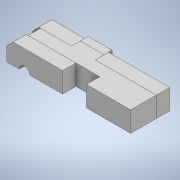
# Autodesk Inventor part: Деталь1
Saved by Autodesk Inventor 2022 (Build 260153000, 153)
## iProperties
Created: 2024-04-16
Part Number: Деталь1
Material: Типовые
Document SubType Name: Modeling
Designer: Pavel
Density: 1 g/cm^3
Appearance: По умолчанию
Mass: 255.555 g
Surface Area: 533.619 cm^2
Volume: 255.555 cm^3
Author: Pavel
Autodesk Inventor part; units mm, degrees
ref_plane "YZ Plane" through (0, 0, 0) normal (1, 0, 0) x (0, 1, 0)
ref_plane "XZ Plane" through (0, 0, 0) normal (0, 1, 0) x (-1, 0, 0)
ref_plane "XY Plane" through (0, 0, 0) normal (0, 0, 1) x (1, 0, 0)
sketch "Эскиз1" plane through (0, 0, 0) normal (0, 1, 0) x (-1, 0, 0)
  line L0 (0, 0) -> (140, 0)
  line L1 (140, 0) -> (140, 46)
  line L2 (140, 46) -> (0, 46)
  line L3 (0, 46) -> (0, 0)
  dimension "d0" = 140
  dimension "d1" = 46
  constraints: 8 end point, 2 parallel, 1 horizontal, 1 perpendicular
  measures "d0" distance of L2.end L1.end
  measures "d1" distance of L1.end L0.end
extrude "Выдавливание1" add sketch "Эскиз1" along normal blind 44
sketch "Эскиз2" plane through (0, 0, 0) normal (0, 0, -1) x (-1, 0, 0)
  line L0 (0, 44) -> (140, 44) projected
  line L1 (0, 44) -> (69, 44)
  line L2 (69, 44) -> (69, 29)
  line L3 (69, 29) -> (0, 29)
  line L4 (0, 29) -> (0, 44)
  point P0 (0, 0)
  dimension "d4" = 69
  dimension "d5" = 15
  constraints: 8 end point, 2 parallel, 1 horizontal, 1 perpendicular
  measures "d4" distance of L2.end L3.end
  measures "d5" distance of L1.end L2.end
split body "Разделение1" sketch "Эскиз2" result two bodies curves L3 L4 L1 L2 first body at (-46.6667, 0.5, 30.6667)
sketch "Эскиз3" plane through (0, 0, 0) normal (0, 0, -1) x (-1, 0, 0)
  line L0 (140, 44) -> (96, 44)
  line L1 (96, 44) -> (96, 29)
  line L2 (96, 29) -> (140, 29)
  line L3 (140, 29) -> (140, 44)
  line L4 (140, 0) -> (77, 0)
  line L5 (77, 0) -> (77, 15)
  line L6 (77, 15) -> (140, 15)
  line L7 (140, 15) -> (140, 0)
  line L8 (77, 0) -> (50, 0)
  line L9 (50, 0) -> (50, 15)
  line L10 (50, 15) -> (77, 15)
  line L11 (77, 15) -> (77, 0)
  point P0 (0, 0)
  dimension "d6" = 44
  dimension "d7" = 15
  dimension "d8" = 63
  dimension "d9" = 15
  dimension "d10" = 27
  dimension "d11" = 15
  constraints: 24 end point, 6 parallel, 3 horizontal, 3 perpendicular, 1 point on line
  measures "d6" distance of L2.end L1.end
  measures "d7" distance of L1.end L0.end
  measures "d8" distance of L5.end L6.end
  measures "d9" distance of L4.end L5.end
  measures "d10" distance of L9.end L10.end
  measures "d11" distance of L8.end L9.end
split body "Разделение2" sketch "Эскиз3" result two bodies bodies 2 curves L1 L2 L3 L0 first body at (-125.3333, 43.5, 30.6667)
sketch "Эскиз4" plane through (0, 0, 0) normal (0, 0, -1) x (-1, 0, 0)
  line L0 (140, 0) -> (140, 29) projected
  line L1 (140, 0) -> (77, 0)
  line L2 (77, 0) -> (77, 15)
  line L3 (77, 15) -> (140, 15)
  line L4 (140, 15) -> (140, 0)
  point P0 (0, 0)
  dimension "d12" = 63
  dimension "d13" = 15
  constraints: 8 end point, 2 parallel, 1 horizontal, 1 perpendicular
  measures "d12" distance of L2.end L3.end
  measures "d13" distance of L1.end L2.end
split body "Разделение3" sketch "Эскиз4" result two bodies bodies 5 curves L1 L2 L3 L4 first body at (-25.6667, 0.5, 30.6667)
sketch "Эскиз5" plane through (0, 29, 0) normal (0, 0, -1) x (-1, 0, 0)
  line L0 (77, -14) -> (77, -29) projected
  line L1 (77, -29) -> (50, -29)
  line L2 (50, -29) -> (50, -14)
  line L3 (50, -14) -> (77, -14)
  line L4 (77, -14) -> (77, -29)
  point P0 (0, -29)
  dimension "d14" = 27
  dimension "d15" = 15
  constraints: 8 end point, 2 parallel, 1 horizontal, 1 perpendicular
  measures "d14" distance of L2.end L3.end
  measures "d15" distance of L1.end L2.end
extrude "Выдавливание2" cut sketch "Эскиз5" against normal blind 51.75 bodies 6
sketch "Эскиз6" plane through (0, 29, 0) normal (0, 0, -1) x (-1, 0, 0)
  line L0 (140, 0) -> (140, 15) projected
  line L1 (140, 0) -> (131, 0)
  line L2 (131, 0) -> (131, -15)
  line L3 (131, -15) -> (140, -15)
  line L4 (140, -15) -> (140, 0)
  point P0 (0, -29)
  dimension "d18" = 9
  dimension "d19" = 15
  constraints: 8 end point, 2 parallel, 1 horizontal, 1 perpendicular
  measures "d18" distance of L3.end L2.end
  measures "d19" distance of L2.end L1.end
extrude "Выдавливание3" cut sketch "Эскиз6" against normal blind 96 bodies 6
chamfer "Фаска1" distance 7 angle 45 4 edges at (-140, 36.5, 0) (-140, 36.5, 46) (-140, 7.5, 0) (-140, 7.5, 46)
sketch "Эскиз7" plane through (0, 44, 0) normal (0, 1, 0) x (1, 0, 0)
  line L0 (-96, 0) -> (-96, -46) projected
  line L1 (-96, -46) -> (-69, -46) projected
  line L2 (-69, 0) -> (-69, -46) projected
  line L3 (-69, 0) -> (-96, 0) projected
  point P0 (0, 0)
extrude "Выдавливание4" add sketch "Эскиз7" along normal blind 4 bodies 6
sketch "Эскиз8" plane through (0, 29, 0) normal (0, 0, -1) x (-1, 0, 0)
  line L0 (69, 19) -> (69, 0) projected
  line L1 (96, 15) -> (96, 0) projected
  line L2 (69, 19) -> (96, 19)
  line L3 (96, 19) -> (96, 10)
  line L4 (96, 10) -> (69, 10)
  line L5 (69, 10) -> (69, 19)
  point P0 (0, -29)
  dimension "d27" = 9
  constraints: 8 end point, 2 parallel, 1 horizontal, 1 perpendicular, 1 point on line
  measures "d27" distance of L2.end L3.end
extrude "Выдавливание5" add sketch "Эскиз8" along normal blind 9 bodies 6
sketch "Эскиз9" plane through (0, 29, -9) normal (0, 0, -1) x (-1, 0, 0)
  line L0 (96, 19) -> (69, 19) projected
  line L1 (69, 19) -> (69, 10) projected
  line L2 (69, 10) -> (96, 10) projected
  line L3 (96, 10) -> (96, 19) projected
  point P0 (0, -29)
split body "Разделение4" sketch "Эскиз9" result two bodies bodies 6 curves L0 L1 L2 L3 first body at (-78, 47.5, 9.3333)
sketch "Эскиз22" plane through (0, 44, 0) normal (0, 1, 0) x (1, 0, 0)
  point P0 (-120, -23)
hole "Отверстие12" at (-120, 44, 23) direction (0, -1, 0) diameter 12 depth 15 bodies 4 clearance for "болты с шестигранной головкой / гайка ГОСТ 12876-67" size "M12" standard "ГОСТ"
sketch "Эскиз23" plane through (-96, 29, 46) normal (0, 1, 0) x (1, 0, 0)
  point P0 (-24, 23)
hole "Отверстие13" at (-120, 29, 23) direction (0, -1, 0) diameter 12 depth 14 bodies 9
sketch "Эскиз24" plane through (0, 0, 0) normal (0, -1, 0) x (1, 0, 0)
  point P0 (-120, 23)
hole "Отверстие14" at (-120, 0, 23) direction (0, 1, 0) diameter 12 depth 15 bodies 7
combine bodies "Комбинировать1" operation type add bodies to combine 7 9
sketch "Эскиз29" plane through (0, 0, 0) normal (0, 0, -1) x (-1, 0, 0)
  line L0 (77, 0) -> (77, 15) projected
  line L1 (140, 0) -> (140, 15) projected
  line L2 (77, 15) -> (140, 15)
  line L3 (140, 15) -> (140, 0)
  line L4 (140, 0) -> (77, 0)
  line L5 (77, 0) -> (77, 15)
  point P0 (0, 0)
  constraints: 8 end point, 2 parallel, 1 horizontal, 1 perpendicular
split body "Разделение5" sketch "Эскиз29" result two bodies bodies 7 curves L2 L3 L4 L5 first body at (-46, 28.5, 30.6667)
sketch "Эскиз34" plane through (0, 44, 0) normal (0, 1, 0) x (1, 0, 0)
  line L0 (0, -46) -> (0, 0) construction
  line L1 (0, -46) -> (-28, -46) construction
  line L2 (-28, -46) -> (-28, -23) construction
  line L3 (0, 0) -> (-69, 0) construction
  circle A0 centre (-28, -23) radius 5 construction
  dimension "d197" = 28
  dimension "d198" = 23
  dimension "d199" = 10
  constraints: 4 end point, 1 centre point, 1 coincident, 1 perpendicular
  measures "d197" distance of L0.start L1.end
  measures "d198" distance of L1.end L2.end
  measures "d199" diameter of A0
hole "Отверстие23" at (-28, 44, 23) direction (0, -1, 0) diameter 10 depth 15 bodies 3
sketch "Эскиз35" plane through (-69, 29, 46) normal (0, 1, 0) x (1, 0, 0)
  circle A0 centre (41, 23) radius 5 projected
  point P0 (69, 46)
hole "Отверстие24" at (-28, 29, 23) direction (0, -1, 0) diameter 8.376 depth 15 tip angle 120 bodies 10 thread size "M10x1.5" class "6H" standard "ISO Metric profile"
sketch "Эскиз36" plane through (0, 48, 0) normal (0, 1, 0) x (1, 0, 0)
  line L0 (-96, -46) -> (-69, -46) construction
  line L1 (-96, -46) -> (-82, -46) construction
  line L2 (-82, -46) -> (-82, -23) construction
  circle A0 centre (-82, -23) radius 7 construction
  point P0 (0, 0)
  dimension "d214" = 14
  dimension "d215" = 23
  dimension "d216" = 14
  constraints: 4 end point, 1 centre point, 1 coincident, 1 perpendicular, 1 point on line
  measures "d214" distance of L0.start L1.end
  measures "d215" distance of L1.end L2.end
  measures "d216" diameter of A0
hole "Отверстие25" at (-82, 48, 23) direction (0, -1, 0) diameter 14 depth 6 bodies 8
sketch "Эскиз37" plane through (-82, 42, 23) normal (0, 1, 0) x (1, 0, 0)
  circle A0 centre (0, 0) radius 7 projected
  point P0 (82, 23)
hole "Отверстие26" at (-82, 42, 23) direction (0, -1, 0) diameter 9 depth 3 bodies 8
sketch "Эскиз38" plane through (-96, 39, 46) normal (0, 1, 0) x (1, 0, 0)
  circle A0 centre (14, 23) radius 4.5 projected
  point P0 (96, 46)
hole "Отверстие27" at (-82, 39, 23) direction (0, -1, 0) diameter 6.647 depth 26 tip angle 120 bodies 11 thread size "M8x1.25" class "6H" standard "ISO Metric profile"
sketch "Эскиз39" plane through (-96, 39, 46) normal (0, 1, 0) x (1, 0, 0)
  circle A0 centre (14, 23) radius 4.5 projected
  point P0 (96, 46)
hole "Отверстие28" at (-82, 39, 23) direction (0, -1, 0) diameter 6.647 depth 26 tip angle 120 bodies 10 thread size "M8x1.25" class "6H" standard "ANSI Metric M Profile"
